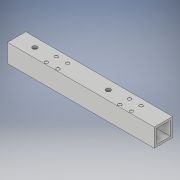
# Autodesk Inventor part: Zero Twosday
Saved by Autodesk Inventor 2018 (Build 220112000, 112)
## iProperties
Created: 2018-12-12
Part Number: Zero Twosday
Material: Generic
Document SubType Name: Modeling
Designer: s-4009421
Density: 1 g/cm^3
Appearance: Default
Author: s-4009421
Autodesk Inventor part; units mm, degrees
ref_plane "YZ Plane" through (0, 0, 0) normal (1, 0, 0) x (0, 1, 0)
ref_plane "XZ Plane" through (0, 0, 0) normal (0, 1, 0) x (-1, 0, 0)
ref_plane "XY Plane" through (0, 0, 0) normal (0, 0, 1) x (1, 0, 0)
sketch "Sketch1" plane through (0, 0, 0) normal (1, 0, 0) x (0, 1, 0)
  line L0 (4.7302, 6.4139) -> (-20.6698, 6.4139)
  line L1 (-20.6698, 6.4139) -> (-20.6698, -18.9861)
  line L2 (-20.6698, -18.9861) -> (4.7302, -18.9861)
  line L3 (4.7302, -18.9861) -> (4.7302, 6.4139)
  line L4 (1.5552, 3.2389) -> (-17.4948, 3.2389)
  line L5 (-17.4948, 3.2389) -> (-17.4948, -15.8111)
  line L6 (-17.4948, -15.8111) -> (1.5552, -15.8111)
  line L7 (1.5552, -15.8111) -> (1.5552, 3.2389)
  point P0 (0, 0)
  dimension "d0" = 25.4
  dimension "d1" = 25.4
  dimension "d2" = 3.175
  constraints: 16 end point, 4 parallel, 2 perpendicular, 1 horizontal, 3 other
  measures "d0" distance of L2.end L1.end
  measures "d1" distance of L1.end L0.end
  measures "d2" distance between parallel lines of L3 L7
extrude "Extrusion1" add sketch "Sketch1" along normal blind 203.2
sketch "Sketch2" plane through (0, 4.7302, 6.4139) normal (0, 1, 0) x (1, 0, 0)
  line L0 (0, 3.175) -> (0, 22.225) projected
  circle A0 centre (25.4, 12.7) radius 3.175
  circle A1 centre (127, 12.7) radius 3.175
  point P0 (0, 6.4139)
  dimension "d6" = 6.35
  dimension "d8" = 6.35
  constraints: 2 centre point
  measures "d6" diameter of A0
  measures "d8" diameter of A1
extrude "Extrusion2" cut sketch "Sketch2" against normal blind 203.2
sketch "Sketch3" plane through (0, 4.7302, 6.4139) normal (0, 1, 0) x (1, 0, 0)
  line L0 (0, 25.4) -> (203.2, 25.4) projected
  line L1 (0, 22.225) -> (0, 3.175) projected
  circle A0 centre (66.802, 16.6589) radius 2.2987
  circle A1 centre (66.802, 3.1715) radius 2.2987
  circle A2 centre (50.8, 3.1715) radius 2.2987
  circle A3 centre (152.4, 16.6589) radius 2.2987
  circle A4 centre (152.4, 3.1715) radius 2.2987
  circle A5 centre (168.402, 3.1715) radius 2.2987
  circle A6 centre (168.402, 16.6589) radius 2.2987
  circle A7 centre (50.8, 16.6589) radius 2.2987
  point P0 (0, 6.4139)
  constraints: 8 centre point
extrude "Extrusion3" cut sketch "Sketch3" against normal blind 0.254
body "Solid1"
